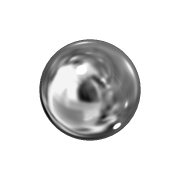
# Autodesk Inventor part: 00_Ballmagnet_5mm
Saved by Autodesk Inventor 2019 (Build 230136000, 136)
## iProperties
Created: 2021-09-23
Part Number: 00_Ballmagnet_5mm
Material: Generisch
Document SubType Name: Modeling
Designer: Muriel
Density: 1 g/cm^3
Appearance: Chrom - poliert
Author: Muriel
Autodesk Inventor part; units mm, degrees
ref_plane "YZ Plane" through (0, 0, 0) normal (1, 0, 0) x (0, 1, 0)
ref_plane "XZ Plane" through (0, 0, 0) normal (0, 1, 0) x (-1, 0, 0)
ref_plane "XY Plane" through (0, 0, 0) normal (0, 0, 1) x (1, 0, 0)
sketch "Skizze1" plane through (0, 0, 0) normal (0, 0, 1) x (1, 0, 0)
  arc A0 (2.45, 0) -> (-2.45, 0) centre (0, 0) ccw
  line L0 (-2.45, 0) -> (2.45, 0)
  dimension "d0" = 2.45
  constraints: 2 end point, 2 point on circle, 1 centre point, 1 coincident, 1 horizontal
  measures "d0" radius of A0
revolve "Umdrehung1" add sketch "Skizze1" angle 360 about axis through (-2.45, 0, 0) along (1, 0, 0)
